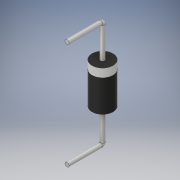
# Autodesk Inventor part: Diode
Saved by Autodesk Inventor 2017 SP1 (Build 210196100, 196)
## iProperties
Part Number: Diode
Material: Generisch
Document SubType Name: Modeling
Designer: Alex
Density: 1 g/cm^3
Appearance: Vorgabe
Author: Alex
Autodesk Inventor part; units mm, degrees
sketch "Skizze3" plane through (0, 0, 0) normal (0, 0, 1) x (1, 0, 0)
  circle A0 centre (0, 0) radius 1.25
  dimension "d0" = 2.5
  constraints: 1 centre point, 1 coincident
  measures "d0" diameter of A0
extrude "Extrusion1" add sketch "Skizze3" along normal blind 4.8
ref_plane "Arbeitsebene1" through (0, 0, 3.8) normal (0, 0, 1) x (1, 0, 0)
split_face "Trennen1"
ref_plane "Arbeitsebene2" through (0, 0, 0) normal (1, 0, 0) x (0, 1, 0)
sketch "Skizze6" plane through (0, 0, 0) normal (1, 0, 0) x (0, 1, 0)
  line L0 (0, 4.8) -> (0, 8.5)
  arc A0 (0, 8.5) -> (-0.25, 8.75) centre (-0.25, 8.5) ccw
  line L1 (-0.25, 8.5) -> (-0.25, 8.75) construction
  line L2 (-0.25, 8.5) -> (0, 8.5) construction
  line L3 (-0.25, 8.75) -> (-4.25, 8.75)
  line L4 (1.25, 4.8) -> (-1.25, 4.8) projected
  line L5 (1.25, 4.8) -> (1.25, 3.8) projected
  line L6 (1.25, 3.8) -> (1.25, 0) projected
  line L7 (1.25, 0) -> (-1.25, 0) projected
  line L8 (-1.25, 0) -> (-1.25, 3.8) projected
  line L9 (-1.25, 3.8) -> (-1.25, 4.8) projected
  line L10 (-1.25, 4.8) -> (1.25, 4.8) projected
  line L11 (-1.25, 3.8) -> (-1.25, 4.8) projected
  point P0 (0, 0)
  dimension "d7" = 90
  dimension "d9" = 3.7
  dimension "d10" = 4
  dimension "d13" = 0.25
  dimension "d20" = 0.25
  dimension "d21" = 1.25
  constraints: 8 end point, 2 point on circle, 1 centre point, 1 coincident, 1 horizontal, 1 midpoint, 1 vertical
  measures "d7" angle of L2 L1
  measures "d9" distance of L0.start L0.end
  measures "d10" distance of L1.end L3.end
  measures "d13" distance of L0.end point (-0.25, 8.5)
  measures "d20" horizontal distance of L0.end L1.end
  measures "d21" distance between parallel lines of L9 L0
sketch "Skizze4" plane through (0, 0, 4.8) normal (0, 0, 1) x (1, 0, 0)
  circle A0 centre (0, 0) radius 0.25
  dimension "d4" = 0.5
  constraints: 1 centre point, 1 coincident
  measures "d4" diameter of A0
sweep "Sweeping1" add profiles "Skizze4" path "Skizze6" path curves L0 A0 L3
ref_plane "Arbeitsebene3" through (0, 0, 2.4) normal (0, 0, -1) x (-1, 0, 0)
mirror "Spiegeln1" about plane through (0, 0, 2.4) normal (0, 0, -1) of "Sweeping1"
